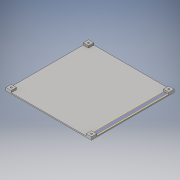
# Autodesk Inventor part: Backplate-housing
Saved by Autodesk Inventor 2016 SP2 (Build 200236200, 236)
## iProperties
Created: 2018-06-21
Part Number: Backplate-housing
Material: Generisch
Document SubType Name: Modeling
Designer: Nils
Density: 1 g/cm^3
Appearance: Vorgabe
Author: Nils
Autodesk Inventor part; units mm, degrees
ref_plane "YZ Plane" through (0, 0, 0) normal (1, 0, 0) x (0, 1, 0)
ref_plane "XZ Plane" through (0, 0, 0) normal (0, 1, 0) x (-1, 0, 0)
ref_plane "XY Plane" through (0, 0, 0) normal (0, 0, 1) x (1, 0, 0)
ref_plane "Arbeitsebene1" through (796.2209, 70.6141, -996.2958) normal (0, 0, -1) x (-1, 0, 0)
sketch "Skizze1" plane through (796.2209, 70.6141, -996.2958) normal (0, 0, -1) x (-1, 0, 0)
  line L0 (-3.9996, -76.75) -> (4.0004, -76.75) construction
  line L1 (-3.9996, 76.75) -> (-3.9996, -76.75) construction
  line L2 (4.0004, 76.75) -> (-3.9996, 76.75) construction
  line L3 (4.0004, 84.25) -> (4.0004, 76.75) construction
  line L4 (-37.8996, 84.25) -> (4.0004, 84.25) construction
  line L5 (-37.8996, 1.75) -> (-37.8996, 84.25) construction
  line L6 (-133.3996, 1.75) -> (-37.8996, 1.75) construction
  line L7 (-133.3996, -84.25) -> (-133.3996, 1.75) construction
  line L8 (4.0004, -84.25) -> (-133.3996, -84.25) construction
  line L9 (4.0004, -76.75) -> (4.0004, -84.25) construction
  line L10 (150.8004, -76.75) -> (142.8004, -76.75) construction
  line L11 (142.8004, -76.75) -> (142.8004, -84.25) construction
  line L12 (142.8004, -84.25) -> (280.2004, -84.25) construction
  line L13 (280.2004, -84.25) -> (280.2004, 1.75) construction
  line L14 (280.2004, 1.75) -> (184.7004, 1.75) construction
  line L15 (184.7004, 1.75) -> (184.7004, 84.25) construction
  line L16 (184.7004, 84.25) -> (142.8004, 84.25) construction
  line L17 (142.8004, 84.25) -> (142.8004, 76.75) construction
  line L18 (142.8004, 76.75) -> (150.8004, 76.75) construction
  line L19 (150.8004, 76.75) -> (150.8004, -76.75) construction
  line L20 (-5.9996, 76.75) -> (-5.9996, -76.75) construction
  line L21 (152.8004, 76.75) -> (152.8004, -76.75) construction
  line L22 (-5.9996, 76.75) -> (152.8004, 76.75) construction
  line L23 (-5.9996, -76.75) -> (152.8004, -76.75) construction
  line L24 (73.4004, -76.75) -> (73.4004, 76.75) construction
  line L25 (-5.8996, -76.65) -> (152.7004, -76.65)
  line L26 (152.7004, -76.65) -> (152.7004, 76.65)
  line L27 (152.7004, 76.65) -> (-5.8996, 76.65)
  line L28 (-5.8996, 76.65) -> (-5.8996, -76.65)
  line L29 (-5.8996, -76.65) -> (152.7004, 76.65) construction
  line L30 (152.7004, -76.65) -> (-5.8996, 76.65) construction
  point P0 (796.2209, -70.6141)
  point P1 (73.4004, 0)
  dimension "d24" = 0.1
  dimension "d25" = 0.1
  constraints: 22 end point, 5 midpoint, 3 parallel, 2 vertical, 1 collinear, 1 horizontal, 1 perpendicular, 4 other
  measures "d24" distance between parallel lines of L22 L27
  measures "d25" distance between parallel lines of L21 L26
extrude "Extrusion1" add sketch "Skizze1" along normal blind 2
sketch "Skizze2" plane through (796.2209, 70.6141, -996.2958) normal (0, 0, 1) x (1, 0, 0)
  line L0 (-152.8004, -76.75) -> (-142.8004, -76.75) construction
  line L1 (-142.8004, -66.75) -> (-152.8004, -66.75) construction
  line L2 (-142.8004, -76.75) -> (-142.8004, -66.75) construction
  line L3 (-152.8004, -66.75) -> (-152.8004, -76.75) construction
  line L4 (-4.0004, -66.75) -> (5.9996, -66.75) construction
  line L5 (-4.0004, -76.75) -> (-4.0004, -66.75) construction
  line L6 (5.9996, -66.75) -> (5.9996, -76.75) construction
  line L7 (5.9996, -76.75) -> (-4.0004, -76.75) construction
  line L8 (-152.8004, 66.75) -> (-142.8004, 66.75) construction
  line L9 (-142.8004, 66.75) -> (-142.8004, 76.75) construction
  line L10 (-142.8004, 76.75) -> (-152.8004, 76.75) construction
  line L11 (-152.8004, 76.75) -> (-152.8004, 66.75) construction
  line L12 (-4.0004, 66.75) -> (-4.0004, 76.75) construction
  line L13 (5.9996, 66.75) -> (-4.0004, 66.75) construction
  line L14 (-4.0004, 76.75) -> (5.9996, 76.75) construction
  line L15 (5.9996, 76.75) -> (5.9996, 66.75) construction
  line L16 (-142.9004, -76.65) -> (-152.7004, -76.65)
  line L17 (-152.7004, -76.65) -> (-152.7004, -66.85)
  line L18 (-152.7004, -66.85) -> (-142.9004, -66.85)
  line L19 (-142.9004, -66.85) -> (-142.9004, -76.65)
  line L20 (5.8996, -76.65) -> (-152.7004, -76.65) projected
  line L21 (5.8996, -76.65) -> (5.8996, -66.85)
  line L22 (5.8996, -66.85) -> (-3.9004, -66.85)
  line L23 (-3.9004, -66.85) -> (-3.9004, -76.65)
  line L24 (-3.9004, -76.65) -> (5.8996, -76.65)
  line L25 (5.8996, 76.65) -> (5.8996, -76.65) projected
  line L26 (-3.9004, 66.85) -> (-3.9004, 76.65)
  line L27 (-3.9004, 76.65) -> (5.8996, 76.65)
  line L28 (5.8996, 76.65) -> (5.8996, 66.85)
  line L29 (5.8996, 66.85) -> (-3.9004, 66.85)
  line L30 (-142.9004, 76.65) -> (-142.9004, 66.85)
  line L31 (-142.9004, 66.85) -> (-152.7004, 66.85)
  line L32 (-152.7004, 66.85) -> (-152.7004, 76.65)
  line L33 (-152.7004, 76.65) -> (-142.9004, 76.65)
  line L34 (-152.7004, 76.65) -> (5.8996, 76.65) projected
  point P0 (-796.2209, -70.6141)
  constraints: 64 end point, 8 horizontal, 8 vertical, 4 collinear, 28 other
extrude "Extrusion2" add sketch "Skizze2" along normal blind 3.5
sketch "Skizze3" plane through (796.2209, 70.6141, -992.7958) normal (0, 0, 1) x (1, 0, 0)
  circle A0 centre (0.9996, 71.75) radius 1.75 construction
  circle A1 centre (0.9996, -71.75) radius 1.75 construction
  circle A2 centre (-147.8004, 71.75) radius 1.75 construction
  circle A3 centre (-147.8004, -71.75) radius 1.75 construction
  line L0 (-142.9004, 66.85) -> (-142.9004, 76.65) projected
  line L1 (-142.9004, 76.65) -> (-152.7004, 76.65) projected
  line L2 (-152.7004, 76.65) -> (-152.7004, 66.85) projected
  line L3 (-152.7004, 66.85) -> (-142.9004, 66.85) projected
  circle A4 centre (-147.8004, 71.75) radius 1.5
  circle A5 centre (1.0996, 71.75) radius 1.5
  circle A6 centre (1.0996, -71.75) radius 1.5
  circle A7 centre (-147.8004, -71.75) radius 1.5
  point P0 (-796.2209, -70.6141)
  constraints: 8 centre point, 16 other
extrude "Extrusion3" cut sketch "Skizze3" against normal blind 15.5 contours A4 | A5 | A6 | A7
sketch "Skizze4" plane through (796.2209, 70.6141, -998.2958) normal (0, 0, -1) x (-1, 0, 0)
  circle A0 centre (147.8004, 71.75) radius 1.5 construction
  circle A1 centre (147.8004, -71.75) radius 1.5 construction
  circle A2 centre (-1.0996, -71.75) radius 1.5 construction
  circle A3 centre (147.8004, -71.75) radius 2.85
  circle A4 centre (-1.0996, -71.75) radius 2.85
  circle A5 centre (147.8004, 71.75) radius 2.85
  circle A6 centre (-1.0996, 71.75) radius 2.85
  circle A7 centre (-1.0996, 71.75) radius 1.5 construction
  point P0 (796.2209, -70.6141)
  dimension "d27" = 5.7
  dimension "d28" = 5.7
  dimension "d29" = 5.7
  dimension "d30" = 5.7
  constraints: 4 centre point, 4 coincident
  measures "d27" diameter of A3
  measures "d28" diameter of A4
  measures "d29" diameter of A5
  measures "d30" diameter of A6
extrude "Extrusion4" cut sketch "Skizze4" against normal blind 3.1
equation "\"d28\" = d27"
equation "\"d29\" = d27"
equation "\"d30\" = d27"
